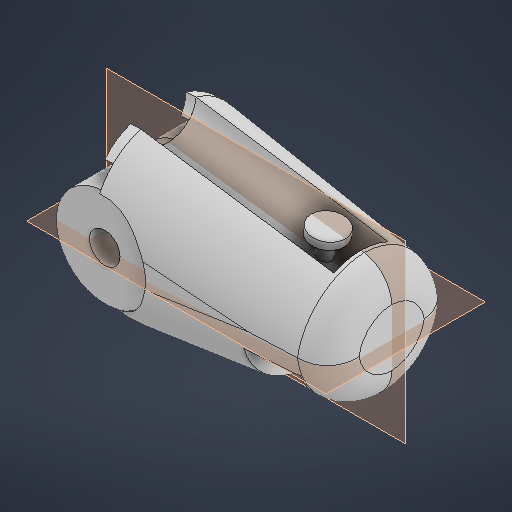
# Autodesk Inventor part: falange3_menique_V12
Saved by Autodesk Inventor 2026.1 (Build 301233020, 233B)
## iProperties
Created: 2026-01-17
Part Number: falange3_menique_V12
Material: Generic
Document SubType Name: Modeling
Designer: user
Density: 1 g/cm^3
Appearance: Default
Author: user
Autodesk Inventor part; units mm, degrees
ref_plane "YZ Plane" through (0, 0, 0) normal (1, 0, 0) x (0, 1, 0)
sketch "Sketch1" plane through (0, 0, 0) normal (0, 0, 1) x (1, 0, 0)
  circle A0 centre (0, 0) radius 1.575
  arc A1 (0, 5) -> (1.3675, -4.8093) centre (0, 0) ccw
  line L0 (0, 5) -> (0, 9)
  line L1 (23, -5.6998) -> (23, 6)
  line L2 (3.4217, -7.743) -> (23, -5.6998)
  line L3 (0, 9) -> (23, 6)
  line L4 (1.3675, -4.8093) -> (3.4217, -7.743)
  line L5 (-11.371, 0) -> (28.7285, 0) projected
  point P0 (23, 0)
  dimension "d0" = 3.15
  dimension "d1" = 10
  dimension "d2" = 4
  dimension "d9" = 23
  dimension "d100" = 55
  dimension "d102" = 9
  constraints: 10 end point, 2 centre point, 2 coincident, 2 point on circle, 2 vertical, 1 parallel, 1 point on line
  measures "d0" diameter of A0
  measures "d1" diameter of A1
  measures "d2" distance of L0.start L0.end
  measures "d9" distance between parallel lines of L1 L0
  measures "d100" angle of L5 L4
  measures "d102" distance of point (0, 0) L0.end
extrude "Extrusion1" add sketch "Sketch1" along normal mid plane 23 contours L5 L1 L2 L4 A1 A0 | A0 L5 A1 L0 L3 L1
sketch "Sketch3" plane through (0, 5, 11.5) normal (-1, 0, 0) x (0, 0, 1)
  circle A0 centre (-11.5, -9.6108) radius 1.5
  point P0 (-11.5, -5)
  dimension "d19" = 3
  constraints: 1 centre point
  measures "d19" diameter of A0
sketch "Sketch5" plane through (0, 0, 11.5) normal (0, 0, 1) x (1, 0, 0)
  line L0 (19.8338, -7.5236) -> (14.4628, -7.5236)
  line L1 (14.4628, -7.5236) -> (14.4628, -1.698)
  line L2 (14.4628, -1.698) -> (19.8338, -1.698)
  line L3 (19.8338, -1.698) -> (19.8338, -7.5236)
  point P0 (0, 0)
  dimension "d24" = 5.8256
  dimension "d28" = 5.3709
  constraints: 8 end point, 2 parallel, 1 horizontal, 1 perpendicular
  measures "d24" distance of L2.end L0.start
  measures "d28" distance of L1.end L2.end
extrude "Extrusion4" cut sketch "Sketch5" against normal through all
sketch "Sketch6" plane through (14.4628, -1.698, 11.5) normal (0, -1, 0) x (1, 0, 0)
  circle A0 centre (2.9263, -11.5) radius 1
  point P0 (-14.4628, -11.5)
  dimension "d33" = 2
  constraints: 1 centre point
  measures "d33" diameter of A0
sketch "Sketch24" plane through (0, 0, 0) normal (0, 1, 0) x (-1, 0, 0)
  line L0 (9.5042, 0) -> (9.5042, -7.7045)
  line L1 (0, -11.5) -> (0, 11.5) projected
  line L2 (9.5042, -7.7045) -> (0, -7.7045)
  line L3 (-23, -11.5) -> (-23, 11.5) projected
  line L4 (0, -7.7045) -> (-23, -6.5)
  line L5 (-23, -6.5) -> (-23, 0)
  line L6 (-23, -6.5) -> (-23, 0)
  line L7 (20.588, 0) -> (-42.8071, 0)
  line L8 (9.5042, 0) -> (9.5042, 7.7045)
  line L9 (9.5042, 7.7045) -> (0, 7.7045)
  line L10 (0, 7.7045) -> (-23, 6.5)
  line L11 (-23, 6.5) -> (-23, 0)
  line L12 (-23, 6.5) -> (-23, 0)
  point P0 (0, 0)
  dimension "d103" = 7.7045
  dimension "d104" = 6.5
  constraints: 22 end point, 3 symmetric about line, 2 point on line, 1 collinear, 1 horizontal, 1 midpoint, 1 perpendicular, 1 vertical
  measures "d103" distance of L0.start L0.end
  measures "d104" distance of L4.end L5.end
extrude "Extrusion21" cut sketch "Sketch24" along normal mid plane 26 keep common part
extrude "Extrusion7" cut sketch "Sketch3" against normal blind 15
fillet "Fillet1" radius 6.7625 2 edges at (11.5, 7.5, 7.1023) (11.5, 7.5, -7.1023)
fillet "Fillet2" radius 6.7625 4 edges at (21.4169, -5.865, -6.5829) (8.9423, -7.1669, -7.2362) (8.9423, -7.1669, 7.2362) (21.4169, -5.865, 6.5829)
fillet "Fillet3" radius 3.2625 4 edges at (23, 4.2573, -4.2835) (23, 4.2573, 4.2835) (23, -3.9563, 4.2835) (23, -3.9563, -4.2835)
sketch "Sketch8" plane through (0, 0, 11.5) normal (0, 0, 1) x (1, 0, 0)
  circle A0 centre (0, 0) radius 5.075
  dimension "d50" = 10.15
  constraints: 1 centre point, 1 coincident
  measures "d50" diameter of A0
sketch "Sketch9" plane through (0, 0, -11.5) normal (0, 0, -1) x (-1, 0, 0)
  circle A0 centre (0, 0) radius 5.075
  dimension "d51" = 10.15
  constraints: 1 centre point, 1 coincident
  measures "d51" diameter of A0
extrude "Extrusion8" cut sketch "Sketch9" against normal blind 4.945
extrude "Extrusion9" cut sketch "Sketch8" against normal blind 4.945
ref_plane "Work Plane1" through (0, 9, -11.5) normal (0, 1, 0) x (-1, 0, 0)
sketch "Sketch14" plane through (0, 0, 0) normal (0, 0, 1) x (1, 0, 0)
  circle A0 centre (0, 0) radius 5
  dimension "d76" = 10
  constraints: 1 centre point, 1 coincident
  measures "d76" diameter of A0
extrude "Extrusion14" cut sketch "Sketch14" along normal mid plane 3.825
sketch "Sketch15" plane through (0, 0, -1.9125) normal (0, 0, 1) x (1, 0, 0)
  point P0 (0, 0)
sketch "Sketch16" plane through (0, 0, 0) normal (0, 0, 1) x (1, 0, 0)
  circle A0 centre (0, 0) radius 1.575 projected
  line L0 (-1.4742, 2.734) -> (1.6306, 2.6437)
  line L1 (1.6306, 2.6437) -> (3.1048, -0.0903)
  line L2 (3.1048, -0.0903) -> (1.4742, -2.734)
  line L3 (1.4742, -2.734) -> (-1.6306, -2.6437)
  line L4 (-1.6306, -2.6437) -> (-3.1048, 0.0903)
  line L5 (-3.1048, 0.0903) -> (-1.4742, 2.734)
  dimension "d75" = 5.38
  constraints: 12 end point, 1 coincident, 13 other
  measures "d75" distance between parallel lines of L3 L0
extrude "Extrusion15" cut sketch "Sketch16" along normal mid plane 8.085 contours A0 | L0 L1 L2 L3 L4 L5
sketch "Sketch18" plane through (0, 9, -11.5) normal (-1, 0, 0) x (0, 0, 1)
  line L0 (0, 0) -> (23, 0) projected
  circle A0 centre (11.5, 0) radius 2.8604
  point P0 (11.5, -9)
  dimension "d82" = 5.7208
  constraints: 1 centre point, 1 midpoint
  measures "d82" diameter of A0
sketch "Sketch19" plane through (0, 9, 11.5) normal (0.1293392, 0.9916004, 0) x (0.9916004, -0.1293392, 0)
  line L0 (0, 23) -> (0, 0) projected
  line L1 (0, 11.5) -> (20, 11.5)
  point P0 (1.1641, 11.5)
  dimension "d83" = 20
  constraints: 2 end point, 1 horizontal, 1 midpoint
  measures "d83" distance of L1.start L1.end
sweep "Sweep1" cut profiles "Sketch18" path "Sketch19" path curves L1
ref_plane "Work Plane3" through (-0.3669, 6.1875, 0) normal (0.1293392, 0.9916004, 0) x (0.9916004, -0.1293392, 0)
sketch "Sketch20" plane through (-0.3669, 6.1875, 0) normal (0.1293392, 0.9916004, 0) x (0.9916004, -0.1293392, 0)
  ellipse E0 centre (0, 0) end of major axis (0, -2.8604) minor radius 0.37 (0.0343, -2.848) -> (0.0343, 2.848) ccw projected
  line L0 (0.37, 0) -> (16.61, 0)
  circle A0 centre (16.61, 0) radius 0.7321
  point P0 (1.1641, 0)
  point P1 (0, -2.8604)
  point P2 (0, 2.8604)
  dimension "d86" = 16.24
  dimension "d87" = 1.4642
  constraints: 2 end point, 1 centre point, 1 coincident, 1 horizontal, 2 other
  measures "d86" distance of L0.start L0.end
  measures "d87" diameter of A0
extrude "Extrusion17" add sketch "Sketch20" along normal mid plane 4.1075
sketch "Sketch21" plane through (16.3692, 6.0756, 0) normal (0.1293392, 0.9916004, 0) x (0.9916004, -0.1293392, 0)
  circle A0 centre (0, 0) radius 1.774
  point P0 (-15.4459, 0)
  dimension "d90" = 3.548
  constraints: 1 centre point
  measures "d90" diameter of A0
extrude "Extrusion18" add sketch "Sketch21" along normal up to surface (0.7826 mm away)
extrude "Extrusion19" add sketch "Sketch6" along normal blind 3.1075
sketch "Sketch22" plane through (19.8338, -5.1662, 11.5) normal (-1, 0, 0) x (0, 0, 1)
  circle A0 centre (-11.5, 1.494) radius 1
  line L0 (-10.5, 3.4682) -> (-10.5, 0.3607) projected
  point P0 (-11.5, 5.1662)
  constraints: 1 centre point, 1 tangent
extrude "Extrusion20" add sketch "Sketch22" along normal up to surface round surface about axis through (17.3891, -1.698, 0) along (0, -1, 0) radius 1 far side no
sketch "Sketch23" plane through (0, 5, -6.555) normal (-1, 0, 0) x (0, 0, 1)
  line L0 (12.2384, 2.0724) -> (8.6707, 2.0607)
  arc A0 (8.6707, 2.0607) -> (9.4043, 3.7341) centre (6.555, 3.9857) ccw
  line L1 (6.555, 4.4704) -> (6.555, 0.3405)
  line L2 (0.8716, 2.0724) -> (4.4393, 2.0607)
  arc A1 (3.7057, 3.7341) -> (4.4393, 2.0607) centre (6.555, 3.9857) ccw
  line L3 (0.055, -5) -> (13.055, -5) projected
  line L4 (0.8802, -5) -> (11.7501, -5)
  ellipse E0 centre (5.6223, -2.8198) end of major axis (3.0779, 3.5175) minor radius 6.7625 (3.707, 3.7344) -> (-0.5285, 0.075) ccw projected
  ellipse E1 centre (7.4877, -2.8198) end of major axis (10.0321, 3.5175) minor radius 6.7625 (13.6385, 0.075) -> (9.403, 3.7344) ccw projected
  point P0 (6.555, -5)
  point P1 (-4.945, -5)
  point P2 (18.055, -5)
  constraints: 8 end point, 2 point on line, 2 vertical, 1 symmetric about line, 14 other
revolve "Revolution1" add sketch "Sketch23" angle 7 about axis through (0, 0, -5.6748) along (0, 0, 1)
equation "\"d0\" = diametroDentroUnion + tolerancia"
equation "\"d1\" = diametroFueraUnion"
equation "\"d50\" = diametroFueraUnion + tolerancia"
equation "\"d51\" = diametroFueraUnion + tolerancia"
equation "\"d76\" = diametroFueraUnion"
equation "\"d10\" = 10.639"
equation "\"d16\" = 135deg"
equation "\"d26\" = 135deg"
equation "\"d27\" = 135deg"
equation "\"d30\" = 135deg"
equation "\"d34\" = 23"
equation "\"d35\" = 0"
equation "\"d40\" = 135deg"
equation "\"d41\" = 10.639"
equation "\"d42\" = 11.8875"
equation "\"d43\" = 0"
equation "\"diametroDentroUnion\" = 3"
equation "\"diametroFueraUnion\" = 10"
equation "\"d45\" = 15"
equation "\"d39\" = diametroDentroUnion"
equation "\"tolerancia\" = 0.15"
body "Solid1"
